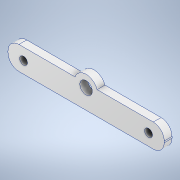
# Autodesk Inventor part: lacznik_pary_kol_V3
Saved by Autodesk Inventor 2020.3 (Build 243373000, 373)
## iProperties
Created: 2021-04-10
Part Number: lacznik_pary_kol_V3
Material: Aluminum 6061
Document SubType Name: Modeling
Designer: patryk.szydlik
Density: 2.7 g/cm^3
Appearance: Aluminum - Flat
Mass: 19.5831 g
Surface Area: 42.4834 cm^2
Volume: 7.25298 cm^3
Author: patryk.szydlik
Autodesk Inventor part; units mm, degrees
ref_plane "YZ Plane" through (0, 0, 0) normal (1, 0, 0) x (0, 1, 0)
ref_plane "XZ Plane" through (0, 0, 0) normal (0, 1, 0) x (-1, 0, 0)
ref_plane "XY Plane" through (0, 0, 0) normal (0, 0, 1) x (1, 0, 0)
sketch "Sketch1" plane through (0, 0, 0) normal (0, 0, 1) x (1, 0, 0)
  line L0 (-1.5978, -2.2765) -> (34.3311, -2.2765)
  line L1 (91.4022, -9.2765) -> (91.4022, -10.2765)
  line L2 (84.4022, -17.2765) -> (-1.5978, -17.2765)
  line L3 (-8.5978, -10.2765) -> (-8.5978, -9.2765)
  arc A0 (-1.5978, -2.2765) -> (-8.5978, -9.2765) centre (-1.5978, -9.2765) ccw
  arc A1 (-8.5978, -10.2765) -> (-1.5978, -17.2765) centre (-1.5978, -10.2765) ccw
  arc A2 (84.4022, -17.2765) -> (91.4022, -10.2765) centre (84.4022, -10.2765) ccw
  arc A3 (91.4022, -9.2765) -> (84.4022, -2.2765) centre (84.4022, -9.2765) ccw
  circle A4 centre (1.4022, -9.7765) radius 2.5
  circle A5 centre (81.4022, -9.7765) radius 2.5
  circle A6 centre (41.4022, -4.7765) radius 4
  arc A7 (48.4732, -2.2765) -> (34.3311, -2.2765) centre (41.4022, -4.7765) ccw
  line L4 (34.3311, -2.2765) -> (48.4732, -2.2765)
  line L5 (48.4732, -2.2765) -> (84.4022, -2.2765)
  arc A8 (34.3311, -2.2765) -> (48.4732, -2.2765) centre (41.4022, -4.7765) ccw
  point P0 (0, 0)
  point P1 (91.4022, -17.2765)
  point P2 (91.4022, -2.2765)
  point P3 (-8.5978, -17.2765)
  point P4 (41.4022, -2.2765)
  dimension "d0" = 100
  dimension "d1" = 15
  dimension "d2" = 7
  dimension "d3" = 5
  dimension "d4" = 5
  dimension "d7" = 8
  dimension "d8" = 7.5
  dimension "d9" = 7.5
  dimension "d10" = 80
  dimension "d11" = 10
  dimension "d13" = 2.5
  dimension "d14" = 40
  dimension "d16" = 15
  constraints: 12 end point, 12 point on circle, 12 tangent, 9 centre point, 7 point on line, 4 parallel, 3 equal radius, 3 horizontal, 3 perpendicular, 2 coincident, 1 horizontal alignment, 1 midpoint, 1 vertical alignment
  measures "d0" distance of point (91.402, -17.277) point (-8.598, -17.277)
  measures "d1" distance of point (91.402, -2.277) point (91.402, -17.277)
  measures "d2" radius of A0
  measures "d3" diameter of A4
  measures "d4" diameter of A5
  measures "d7" diameter of A6
  measures "d8" distance from line of L0 A4.centre
  measures "d9" distance from line of L0 A5.centre
  measures "d10" distance of A5.centre A4.centre
  measures "d11" distance from line of L1 A5.centre
  measures "d13" distance from line of L0 A6.centre
  measures "d14" horizontal distance of A5.centre point (41.402, -4.777)
  measures "d16" diameter of A7
extrude "Extrusion1" add sketch "Sketch1" along normal blind 5 contours L0 A8 L5 A3 L1 A2 L2 A1 L3 A0 | A7 L4 A6 | L4 A6 A8
equation "\"d8\" = 0.5 * d1"
body "Solid1"
